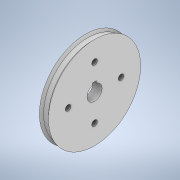
# Autodesk Inventor part: polea sesion 2
Saved by Autodesk Inventor 2022 (Build 260153000, 153)
## iProperties
Created: 2024-02-06
Part Number: polea sesion 2
Material: Generic
Document SubType Name: Modeling
Designer: HP15BW010LA
Density: 1 g/cm^3
Appearance: Default
Author: HP15BW010LA
Autodesk Inventor part; units mm, degrees
ref_plane "YZ Plane" through (0, 0, 0) normal (1, 0, 0) x (0, 1, 0)
ref_plane "XZ Plane" through (0, 0, 0) normal (0, 1, 0) x (-1, 0, 0)
ref_plane "XY Plane" through (0, 0, 0) normal (0, 0, 1) x (1, 0, 0)
sketch "Sketch1" plane through (0, 0, 0) normal (0, 0, 1) x (1, 0, 0)
  line L0 (50, 250) -> (50, -250)
  line L1 (50, -250) -> (-50, -250)
  line L2 (-50, -250) -> (-50, 250)
  line L3 (-50, 250) -> (50, -250) construction
  line L4 (50, 250) -> (-50, -250) construction
  line L5 (-50, 250) -> (-32.3223, 232.3223)
  line L6 (50, 250) -> (32.3223, 232.3223)
  line L7 (-32.3223, 232.3223) -> (32.3223, 232.3223)
  line L8 (0, -350) -> (-200, -350)
  point P0 (0, 0)
  constraints: 18 end point, 2 midpoint, 1 horizontal, 1 parallel
revolve "Revolution1" add sketch "Sketch1" angle 360 about axis through (0, -350, 0) along (-1, 0, 0)
sketch "Sketch2" plane through (50, -350, 0) normal (1, 0, 0) x (0, 0, -1)
  circle A0 centre (0, 350) radius 37.5
  circle A1 centre (0, 0) radius 350
  circle A2 centre (-350, 0) radius 37.5
  circle A3 centre (0, 0) radius 350
  circle A4 centre (0, -350) radius 37.5
  circle A5 centre (0, 0) radius 350
  circle A6 centre (350, 0) radius 37.5
  circle A7 centre (0, 0) radius 350
  dimension "d12" = 360
  constraints: 4 centre point, 3 coincident, 2 horizontal alignment, 2 vertical alignment, 23 other
extrude "Extrusion1" cut sketch "Sketch2" against normal through all contours A0 A1 | A1 A0 | A2 A1 | A1 A2 | A6 A1 | A1 A6 | A4 A1 | A1 A4
thicken "Thicken1" operation add thickness 10 both sides no extend neighbours yes toward (1, 0, 0) faces at (50, -614.9419, 262.9039)
thicken "Thicken2" operation add thickness 10 both sides no extend neighbours yes toward (-1, 0, 0) faces at (-50, -614.9419, 262.9039)
sketch "Sketch3" plane through (60, -350, 0) normal (1, 0, 0) x (0, 0, -1)
  line L0 (-25, 125) -> (25, 125)
  line L1 (25, 125) -> (25, 96.8246)
  line L2 (-25, 96.8246) -> (-25, 125)
  circle A0 centre (0, 0) radius 100 projected
  line L3 (-25, 125) -> (0, 100) construction
  line L4 (25, 125) -> (0, 100) construction
  circle A1 centre (0, 0) radius 100
  point P0 (0, 350)
  constraints: 10 end point, 3 point on circle, 1 centre point, 1 coincident, 1 horizontal, 1 parallel, 1 perpendicular, 3 other
extrude "Extrusion2" cut sketch "Sketch3" along normal through all both and the other way through all contours L0 L1 A0 L2
body "Solid1"
